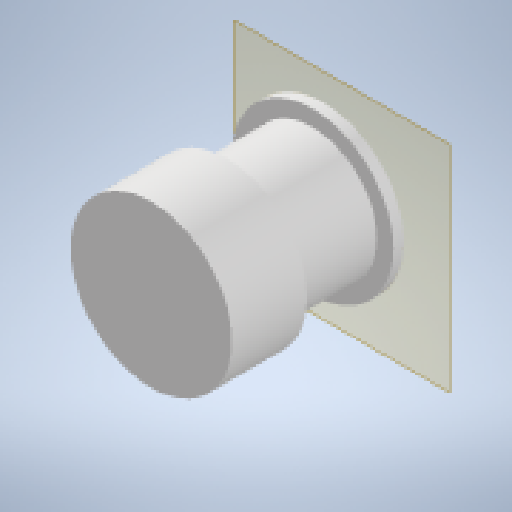
# Autodesk Inventor part: small pulley
Saved by Autodesk Inventor 2024 (Build 280153000, 153)
## iProperties
Created: 2024-04-09
Part Number: small pulley
Material: Generic
Document SubType Name: Modeling
Designer: drew
Density: 1 g/cm^3
Appearance: Default
Author: drew
Autodesk Inventor part; units mm, degrees
ref_plane "YZ Plane" through (0, 0, 0) normal (1, 0, 0) x (0, 1, 0)
ref_plane "XZ Plane" through (0, 0, 0) normal (0, 1, 0) x (-1, 0, 0)
ref_plane "Work Plane1" through (0, 0, -20) normal (0, 0, 1) x (1, 0, 0)
sketch "Sketch1" plane through (0, 0, -20) normal (0, 0, 1) x (1, 0, 0)
  circle A0 centre (-1.75, 0) radius 15.5 projected
  circle A1 centre (-1.75, 0) radius 7.5
  point P0 (0, 0)
  dimension "d1" = 15
  constraints: 1 centre point, 1 coincident
  measures "d1" diameter of A1
extrude "Extrusion1" add sketch "Sketch1" along normal blind 1 contours A1
sketch "Sketch2" plane through (-1.75, 0, -19) normal (0, 0, 1) x (1, 0, 0)
  circle A0 centre (0, 0) radius 7.5 projected
  circle A1 centre (0, 0) radius 6
  point P0 (1.75, 0)
  dimension "d4" = 12
  constraints: 1 centre point, 1 coincident
  measures "d4" diameter of A1
extrude "Extrusion2" add sketch "Sketch2" along normal blind 8 contours A1
sketch "Sketch3" plane through (-1.75, 0, -11) normal (0, 0, 1) x (1, 0, 0)
  circle A0 centre (0, 0) radius 7.5 projected
  circle A1 centre (0, 0) radius 7.5
  point P0 (1.75, 0)
  constraints: 1 centre point, 1 coincident, 1 concentric
extrude "Extrusion3" add sketch "Sketch3" along normal blind 7
body "Solid1"
